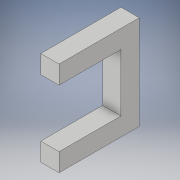
# Autodesk Inventor part: Main
Saved by Autodesk Inventor 2019 (Build 230136000, 136)
## iProperties
Created: 2018-08-02
Part Number: Main
Material: Generic
Document SubType Name: Modeling
Designer: zacha
Density: 1 g/cm^3
Appearance: Default
Author: zacha
Autodesk Inventor part; units mm, degrees
ref_plane "YZ Plane" through (0, 0, 0) normal (1, 0, 0) x (0, 1, 0)
ref_plane "XZ Plane" through (0, 0, 0) normal (0, 1, 0) x (-1, 0, 0)
ref_plane "XY Plane" through (0, 0, 0) normal (0, 0, 1) x (1, 0, 0)
sketch "Sketch1" plane through (0, 0, 0) normal (1, 0, 0) x (0, 1, 0)
  line L0 (0, 0) -> (20, 0) construction
  line L1 (20, 0) -> (20, -21.5)
  line L2 (20, -21.5) -> (0, -21.5)
  line L3 (0, -21.5) -> (0, 0)
  line L4 (20, 0) -> (26.35, 0)
  line L5 (26.35, 0) -> (26.35, -27.85)
  line L6 (-6.35, -27.85) -> (-6.35, 0)
  line L7 (-6.35, 0) -> (0, 0)
  line L8 (26.35, -27.85) -> (-6.35, -27.85)
  dimension "d0" = 20
  dimension "d1" = 21.5
  dimension "d4" = 6.35
  dimension "d23" = 6.35
  dimension "d24" = 6.35
  constraints: 18 end point, 3 horizontal, 3 perpendicular, 2 parallel
  measures "d0" distance of L1.end L2.end
  measures "d1" distance of L0.end L1.end
  measures "d4" distance between parallel lines of L6 L3
  measures "d23" distance of L0.end L4.end
  measures "d24" distance between parallel lines of L8 L2
extrude "Extrusion1" add sketch "Sketch1" along normal blind 6.35
body "Solid1"
